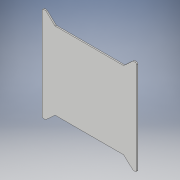
# Autodesk Inventor part: New Plate
Saved by Autodesk Inventor 2017 (Build 210142000, 142)
## iProperties
Created: 2017-03-05
Part Number: New Plate
Material: Generic
Document SubType Name: Modeling
Designer: gilef
Density: 1 g/cm^3
Appearance: Default
Author: gilef
Autodesk Inventor part; units mm, degrees
ref_plane "YZ Plane" through (0, 0, 0) normal (1, 0, 0) x (0, 1, 0)
ref_plane "XZ Plane" through (0, 0, 0) normal (0, 1, 0) x (-1, 0, 0)
ref_plane "XY Plane" through (0, 0, 0) normal (0, 0, 1) x (1, 0, 0)
sketch "Sketch1" plane through (0, 0, 0) normal (0, 0, 1) x (1, 0, 0)
  line L0 (0, 0) -> (218, 0)
  line L1 (218, 0) -> (218, 218)
  line L2 (218, 218) -> (0, 218)
  line L3 (0, 218) -> (0, 0)
  dimension "d0" = 218
  dimension "d1" = 218
  constraints: 8 end point, 2 parallel, 1 horizontal, 1 perpendicular
  measures "d0" distance of L1.end L2.end
  measures "d1" distance of L0.end L1.end
extrude "Extrusion1" add sketch "Sketch1" along normal blind 3
fillet "Fillet1" radius 3.175 4 edges at (218, 0, 1.5) (218, 218, 1.5) (0, 218, 1.5) (0, 0, 1.5)
sketch "Sketch2" plane through (0, 0, 3) normal (0, 0, 1) x (1, 0, 0)
  arc A0 (0, 3.175) -> (3.175, 0) centre (3.175, 3.175) ccw projected
  line L0 (3.175, 0) -> (214.825, 0) projected
  arc A1 (214.825, 0) -> (218, 3.175) centre (214.825, 3.175) ccw projected
  line L1 (218, 3.175) -> (218, 214.825) projected
  arc A2 (218, 214.825) -> (214.825, 218) centre (214.825, 214.825) ccw projected
  line L2 (214.825, 218) -> (3.175, 218) projected
  arc A3 (3.175, 218) -> (0, 214.825) centre (3.175, 214.825) ccw projected
  line L3 (0, 214.825) -> (0, 3.175) projected
  line L4 (214.825, 218) -> (3.175, 218) projected
  line L5 (30, 198) -> (188, 198)
  line L6 (3.175, 218) -> (8.175, 218)
  line L7 (8.175, 218) -> (30, 198)
  line L8 (214.825, 218) -> (209.825, 218)
  line L9 (188, 198) -> (209.825, 218)
  line L10 (0, 214.825) -> (0, 3.175) construction
  line L11 (0, 109) -> (218, 109) construction
  line L12 (30, 20) -> (188, 20)
  line L13 (3.175, 0) -> (8.175, 0)
  line L14 (8.175, 0) -> (30, 20)
  line L15 (214.825, 0) -> (209.825, 0)
  line L16 (188, 20) -> (209.825, 0)
  point P0 (0, 0)
  point P1 (5.675, 218)
  point P2 (212.325, 218)
  dimension "d5" = 20
  dimension "d6" = 30
  dimension "d7" = 30
  dimension "d8" = 20
  dimension "d9" = 5
  dimension "d10" = 5
  constraints: 22 end point, 4 midpoint, 4 symmetric about line, 2 horizontal alignment
  measures "d5" distance from line of L2 L5.start
  measures "d6" distance from line of L3 L5.start
  measures "d7" distance from line of L1 L5.end
  measures "d8" distance from line of L2 L5.end
  measures "d9" distance of L2.end L6.end
  measures "d10" distance of L2.start L8.end
extrude "Extrusion2" cut sketch "Sketch2" against normal through all contours L14 L12 L16 L0 | L2 L9 L5 L7
body "Solid1"
